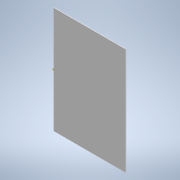
# Autodesk Inventor part: capot
Saved by Autodesk Inventor 2022 (Build 260153000, 153)
## iProperties
Created: 2022-08-02
Part Number: capot
Material: Generic
Document SubType Name: Modeling
Designer: thoma
Density: 1 g/cm^3
Appearance: Default
Author: thoma
Autodesk Inventor part; units mm, degrees
ref_plane "YZ Plane" through (0, 0, 0) normal (1, 0, 0) x (0, 1, 0)
ref_plane "XZ Plane" through (0, 0, 0) normal (0, 1, 0) x (-1, 0, 0)
ref_plane "XY Plane" through (0, 0, 0) normal (0, 0, 1) x (1, 0, 0)
sketch "Sketch1" plane through (0, 0, 0) normal (0, 0, 1) x (1, 0, 0)
  line L0 (0, 0) -> (-672.6812, 0)
  line L1 (-672.6812, 0) -> (-672.6812, -1000)
  line L2 (-672.6812, -1000) -> (0, -1000)
  line L3 (0, -1000) -> (0, 0)
  constraints: 8 end point, 2 parallel, 2 point on line, 1 horizontal, 1 perpendicular, 1 other
extrude "Extrusion1" add sketch "Sketch1" along normal blind 6
body "Solid1"
